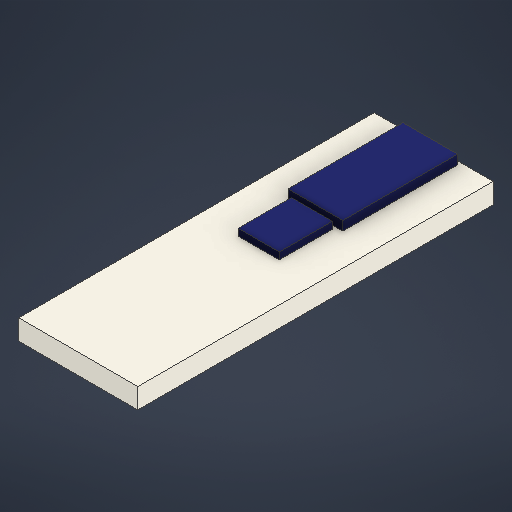
# Autodesk Inventor part: Breadboard
Saved by Autodesk Inventor 2025 (Build 290162000, 162)
## iProperties
Created: 2024-04-22
Part Number: Breadboard
Material: Generic
Document SubType Name: Modeling
Designer: conno
Density: 1 g/cm^3
Appearance: Default
BreadboardWidth: 2.177 in
BreadboardLength: 6.500 in
BreadboardHeight: 0.370 in
Author: conno
Autodesk Inventor part; units mm, degrees
ref_plane "YZ Plane" through (0, 0, 0) normal (1, 0, 0) x (0, 1, 0)
ref_plane "XZ Plane" through (0, 0, 0) normal (0, 1, 0) x (-1, 0, 0)
ref_plane "XY Plane" through (0, 0, 0) normal (0, 0, 1) x (1, 0, 0)
sketch "Sketch1" plane through (0, 0, 0) normal (0, 1, 0) x (-1, 0, 0)
  line L0 (-27.6479, 82.55) -> (27.6479, 82.55)
  line L1 (27.6479, 82.55) -> (27.6479, -82.55)
  line L2 (27.6479, -82.55) -> (-27.6479, -82.55)
  line L3 (-27.6479, -82.55) -> (-27.6479, 82.55)
  line L4 (-27.6479, 82.55) -> (27.6479, -82.55) construction
  line L5 (27.6479, 82.55) -> (-27.6479, -82.55) construction
  point P0 (0, 0)
  dimension "BreadboardWidth" = 55.2958
  dimension "BreadboardLength" = 165.1
  constraints: 12 end point, 2 midpoint, 2 parallel, 1 horizontal, 1 perpendicular
  measures "BreadboardWidth" distance of L1.end L2.end
  measures "BreadboardLength" distance of L2.end L0.start
extrude "Breadboard" add sketch "Sketch1" along normal mid plane 9.398
sketch "Sketch2" plane through (0, 4.699, 0) normal (0, 1, 0) x (1, 0, 0)
  line L0 (12.7, 27.6225) -> (-12.7, 27.6225)
  line L1 (-12.7, 27.6225) -> (-12.7, 80.9625)
  line L2 (-12.7, 80.9625) -> (12.7, 80.9625)
  line L3 (12.7, 80.9625) -> (12.7, 27.6225)
  line L4 (12.7, 27.6225) -> (-12.7, 80.9625) construction
  line L5 (-12.7, 27.6225) -> (12.7, 80.9625) construction
  line L6 (27.6479, 82.55) -> (-27.6479, 82.55) projected
  point P0 (0, 0)
  point P1 (0, 54.2925)
  dimension "d4" = 25.4
  dimension "d5" = 53.34
  dimension "d6" = 1.5875
  constraints: 12 end point, 2 midpoint, 2 parallel, 1 horizontal, 1 perpendicular, 1 vertical alignment
  measures "d4" distance of L1.end L2.end
  measures "d5" distance of L0.end L1.end
  measures "d6" distance between parallel lines of L6 L2
extrude "mBed" add sketch "Sketch2" along normal blind 4.2672
sketch "Sketch3" plane through (0, 4.699, 0) normal (0, 1, 0) x (1, 0, 0)
  line L0 (9.525, 1.27) -> (-9.525, 1.27)
  line L1 (-9.525, 1.27) -> (-9.525, 26.035)
  line L2 (-9.525, 26.035) -> (9.525, 26.035)
  line L3 (9.525, 26.035) -> (9.525, 1.27)
  line L4 (9.525, 1.27) -> (-9.525, 26.035) construction
  line L5 (-9.525, 1.27) -> (9.525, 26.035) construction
  line L6 (-12.7, 27.6225) -> (12.7, 27.6225) projected
  point P0 (0, 0)
  point P1 (0, 13.6525)
  dimension "d9" = 19.05
  dimension "d10" = 24.765
  dimension "d11" = 1.5875
  constraints: 12 end point, 2 midpoint, 2 parallel, 1 horizontal, 1 perpendicular, 1 vertical alignment
  measures "d9" distance of L1.end L2.end
  measures "d10" distance of L0.end L1.end
  measures "d11" distance between parallel lines of L6 L2
extrude "Bluetooth Chip" add sketch "Sketch3" along normal blind 3.175
body "Solid1"
